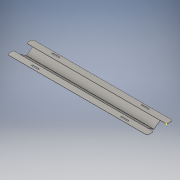
# Autodesk Inventor part: Control pipe holder V2
Saved by Autodesk Inventor 2016 (Build 200138000, 138)
## iProperties
Created: 2017-02-03
Part Number: Control pipe holder V2
Material: Stainless Steel
Document SubType Name: Sheet Metal
Designer: Student
Density: 8 g/cm^3
Flat Pattern Width: 11.2558 cm
Flat Pattern Length: 55.88 cm
Flat Pattern Area: 628.975 cm^2
Sheet Metal Rule: steel noah
Sheet Metal Width: 4.431 in
Sheet Metal Length: 22.000 in
Sheet Metal Area: 97.491 in^2
Appearance: Semi-Polished
Author: Student
Autodesk Inventor part; units mm, degrees
ref_plane "YZ Plane" through (0, 0, 0) normal (1, 0, 0) x (0, 1, 0)
ref_plane "XZ Plane" through (0, 0, 0) normal (0, 1, 0) x (-1, 0, 0)
ref_plane "XY Plane" through (0, 0, 0) normal (0, 0, 1) x (1, 0, 0)
sketch "Sketch1" plane through (0, 0, 0) normal (0, 1, 0) x (-1, 0, 0)
  line L0 (0, 0) -> (0, -25.4)
  line L1 (0, -25.4) -> (558.8, -25.4)
  line L2 (558.8, -25.4) -> (558.8, 0)
  line L3 (558.8, 0) -> (0, 0)
  dimension "d0" = 25.4
  dimension "d1" = 558.8
  measures "d0" distance of L0.start L0.end
  measures "d1" distance of L0.end L1.end
extrude "Plate1" add sketch "Sketch1" along normal blind 0.9652
sketch "Sketch2" plane through (-558.8, 0.1746, -0.5536) normal (0, 0.819152, 0.5735764) x (-1, 0, 0)
  line L0 (-558.8, 0) -> (0, 0)
  line L1 (0, 0) -> (0, 31.75)
  line L2 (0, 31.75) -> (-558.8, 31.75)
  line L3 (-558.8, 31.75) -> (-558.8, 0)
  constraints: 6 end point, 1 horizontal, 1 perpendicular, 1 vertical
edge flange "Flange1" height 31.75 angle 35 thickness 0.9652 bend radius 0.9652 thickness toward (0, 0.819152, 0.5735764) relief tear relief width 0.9652 relief depth 0.4826 edges at (-279.4, 0, 0) wall of the first edge with corners at (0, 0.1746, -0.5536) (-558.8, 0.1746, -0.5536) (-558.8, -18.0365, 25.4545) (0, -18.0365, 25.4545)
bend "Bend1"
corner "Corner1"
sketch "Sketch3" plane through (0, -17.2459, 24.9008) normal (0, -0.819152, 0.5735764) x (1, 0, 0)
  line L0 (-558.8, 0) -> (0, 0)
  line L1 (0, 0) -> (0, 31.75)
  line L2 (0, 31.75) -> (-558.8, 31.75)
  line L3 (-558.8, 31.75) -> (-558.8, 0)
  constraints: 6 end point, 1 horizontal, 1 perpendicular, 1 vertical
edge flange "Flange2" height 31.75 angle 70 thickness 0.9652 bend radius 0.9652 thickness toward (0, -0.819152, 0.5735764) relief tear relief width 0.9652 relief depth 0.4826 edges at (-279.4, -17.2459, 26.0081) wall of the first edge with corners at (-558.8, -17.2459, 24.9008) (0, -17.2459, 24.9008) (0, 0.9652, 50.9089) (-558.8, 0.9652, 50.9089)
bend "Bend2"
corner "Corner2"
sketch "Sketch4" plane through (-558.8, 0, 50.9089) normal (0, 1, 0) x (-1, 0, 0)
  line L0 (-558.8, 0) -> (0, 0)
  line L1 (0, 0) -> (0, 25.4)
  line L2 (0, 25.4) -> (-558.8, 25.4)
  line L3 (-558.8, 25.4) -> (-558.8, 0)
  constraints: 6 end point, 1 horizontal, 1 perpendicular, 1 vertical
edge flange "Flange3" height 25.4 angle 35 thickness 0.9652 bend radius 0.9652 thickness toward (0, 1, 0) relief tear relief width 0.9652 relief depth 0.4826 edges at (-279.4, 0.1746, 51.4625) wall of the first edge with corners at (0, 0, 50.9089) (-558.8, 0, 50.9089) (-558.8, 0, 76.3089) (0, 0, 76.3089)
bend "Bend3"
corner "Corner3"
sketch "Sketch5" plane through (0, 0.9652, 0) normal (0, 1, 0) x (1, 0, 0)
  line L0 (0, -51.5176) -> (-25.4, -51.5176)
  line L1 (0, -51.5176) -> (0, -50.4103) projected
  line L2 (0, -51.5176) -> (0, 0.6087)
  line L3 (0, 0.6087) -> (-25.4, 0.6087)
  line L4 (-25.4, 0.6087) -> (-25.4, -51.5176)
  line L5 (-114.3, -65.0679) -> (-88.9, -65.0679) construction
  line L6 (-114.3, -67.6079) -> (-88.9, -67.6079)
  line L7 (-88.9, -62.5279) -> (-114.3, -62.5279)
  arc A0 (-114.3, -62.5279) -> (-114.3, -67.6079) centre (-114.3, -65.0679) ccw
  arc A1 (-88.9, -67.6079) -> (-88.9, -62.5279) centre (-88.9, -65.0679) ccw
  line L8 (-87.7062, -24.2598) -> (31.8104, -24.2598) construction
  line L9 (-114.3, 19.0882) -> (-88.9, 19.0882)
  line L10 (-88.9, 14.0082) -> (-114.3, 14.0082)
  arc A2 (-114.3, 19.0882) -> (-114.3, 14.0082) centre (-114.3, 16.5482) ccw
  arc A3 (-88.9, 14.0082) -> (-88.9, 19.0882) centre (-88.9, 16.5482) ccw
  line L11 (0, -76.3089) -> (-558.8, -76.3089) projected
  line L12 (-279.4, -268.3812) -> (-279.4, 122.1946) construction
  line L13 (-558.8, -51.5176) -> (-533.4, -51.5176)
  line L14 (-558.8, -51.5176) -> (-558.8, 0.6087)
  line L15 (-558.8, 0.6087) -> (-533.4, 0.6087)
  line L16 (-533.4, 0.6087) -> (-533.4, -51.5176)
  line L17 (-444.5, -67.6079) -> (-469.9, -67.6079)
  line L18 (-469.9, -62.5279) -> (-444.5, -62.5279)
  arc A4 (-444.5, -67.6079) -> (-444.5, -62.5279) centre (-444.5, -65.0679) ccw
  arc A5 (-469.9, -62.5279) -> (-469.9, -67.6079) centre (-469.9, -65.0679) ccw
  line L19 (-469.9, 14.0082) -> (-444.5, 14.0082)
  arc A6 (-444.5, 14.0082) -> (-444.5, 19.0882) centre (-444.5, 16.5482) ccw
  line L20 (-444.5, 19.0882) -> (-469.9, 19.0882)
  arc A7 (-469.9, 19.0882) -> (-469.9, 14.0082) centre (-469.9, 16.5482) ccw
  line L21 (0, -51.5176) -> (0, -76.3089) projected
  point P0 (0, 0)
  point P1 (-101.6, -65.0679)
  point P2 (-457.2, -65.0679)
  dimension "d36" = 25.4
  dimension "d37" = 25.4
  dimension "d38" = 5.08
  dimension "d41" = 88.9
  constraints: 40 end point, 23 symmetric about line, 16 point on circle, 8 centre point, 4 tangent, 2 horizontal, 2 vertical, 1 midpoint, 1 parallel, 1 perpendicular, 6 other
  measures "d36" distance of L2.end L3.end
  measures "d37" distance of L5.start L5.end
  measures "d38" diameter of A1
  measures "d41" distance from line of L21 L5.end
extrude "Cut1" cut sketch "Sketch5" against normal up to next
fillet "Corner Round1" radius 6.35 4 edges at (0, 0.4826, -25.4) (-558.8, 0.4826, 76.3089) (-558.8, 0.4826, -25.4) (0, 0.4826, 76.3089)
fillet "Corner Round2" radius 3.81 4 edges at (-558.8, 0.4826, 51.5176) (0, 0.4826, -0.6087) (0, 0.4826, 51.5176) (-558.8, 0.4826, -0.6087)
sketch "Sketch6" plane through (-533.4, 0.9652, 51.5176) normal (0, 1, 0) x (1, 0, 0)
  point P0 (533.4, 51.5176)
equation "\"d39\" = Thickness"
equation "\"d3\" = BendReliefWidth"
equation "\"d4\" = BendReliefDepth"
equation "\"d5\" = MinimumRemnant"
equation "\"d6\" = BendRadius"
equation "\"d9\" = BendRadius"
equation "\"d10\" = CornerReliefSize"
equation "\"d11\" = GapSize"
equation "\"d12\" = JacobiRadiusSize"
equation "\"d13\" = BendReliefWidth"
equation "\"d14\" = BendReliefDepth"
equation "\"d15\" = MinimumRemnant"
equation "\"d16\" = BendRadius"
equation "\"d19\" = BendRadius"
equation "\"d20\" = CornerReliefSize"
equation "\"d21\" = GapSize"
equation "\"d22\" = JacobiRadiusSize"
equation "\"d23\" = BendReliefWidth"
equation "\"d24\" = BendReliefDepth"
equation "\"d25\" = MinimumRemnant"
equation "\"d26\" = BendRadius"
equation "\"d29\" = BendRadius"
equation "\"d30\" = CornerReliefSize"
equation "\"d31\" = GapSize"
equation "\"d32\" = JacobiRadiusSize"
equation "\"BendRadius\" = Thickness"
equation "\"BendReliefWidth\" = Thickness"
equation "\"BendReliefDepth\" = 0.5 * Thickness"
equation "\"CornerReliefSize\" = 4 * Thickness"
equation "\"MinimumRemnant\" = 2 * Thickness"
equation "\"TransitionRadius\" = BendRadius"
equation "\"JacobiRadiusSize\" = BendRadius"
equation "\"GapSize\" = Thickness"
equation "\"d2\" = BendRadius"
equation "\"Thickness\" = 0.9652"
body "Solid1"
